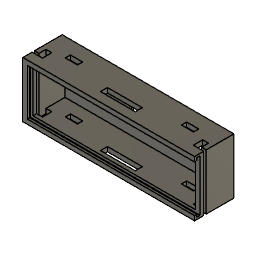
Canal - base v15 (Autodesk Fusion 360 design; units mm, degrees)
Autodesk Fusion 360 part; units mm, degrees
sketch "Esquisse1" plane through (0, 0, 0) normal (0, 1, 0) x (1, 0, 0)
  line L0 (-28.0113, -0.0987) -> (45.9887, -0.0987)
  line L1 (45.9887, -0.0987) -> (45.9887, -24.0987)
  line L2 (45.9887, -24.0987) -> (-28.0113, -24.0987)
  line L3 (-28.0113, -24.0987) -> (-28.0113, -0.0987)
  dimension "d1" = 74
  dimension "d2" = 24
  constraint horizontal L0
  constraint vertical L1
  constraint horizontal L2
  constraint vertical L3
  measures "d1" distance of L1 L3
  measures "d2" distance of L0 L2
extrude "Extrusion1" add sketch "Esquisse1" along normal blind 17
shell "Coque2" thickness 2 removed faces 1 at (21.3221, 0, 16.0987)
sketch "Esquisse3" plane through (0, 0, 0.0987) normal (0, 0, -1) x (1, 0, 0)
  line L0 (45.9887, 0) -> (-28.0113, 0)
  line L1 (-28.0113, 0) -> (-28.0113, -17)
  line L2 (-28.0113, -17) -> (45.9887, -17)
  line L3 (45.9887, -17) -> (45.9887, 0)
  line L4 (16.4887, -7) -> (1.4887, -7)
  line L5 (1.4887, -7) -> (1.4887, -4)
  line L6 (1.4887, -4) -> (16.4887, -4)
  line L7 (16.4887, -4) -> (16.4887, -7)
  line L8 (8.9887, -17) -> (8.9887, 0) construction
  dimension "d12" = 3
  dimension "d14" = 15
  dimension "d15" = 4
  constraint horizontal L4
  constraint vertical L5
  constraint horizontal L6
  constraint vertical L7
  constraint midpoint L2 L8.start
  constraint midpoint L0 L8.end
  constraint symmetric L5 L7 L8
  measures "d12" distance of L4 L6
  measures "d14" distance of L5 L7
  measures "d15" distance of L0 L6
extrude "Extrusion3" cut sketch "Esquisse3" against normal blind 25 contours L4 L5 L6 L7
sketch "Esquisse4" plane through (0, 0, 0) normal (0, 0, 1) x (1, 0, 0)
sketch "Esquisse8" plane through (0, 15, 0) normal (0, -1, 0) x (1, 0, 0)
  line L0 (43.9887, 22.0987) -> (-26.0113, 22.0987)
  line L1 (-26.0113, 22.0987) -> (-26.0113, 2.0987)
  line L2 (-26.0113, 2.0987) -> (43.9887, 2.0987)
  line L3 (43.9887, 2.0987) -> (43.9887, 22.0987)
  line L4 (-26.0113, 22.0987) -> (43.9887, 22.0987)
  line L5 (43.9887, 22.0987) -> (43.9887, 2.0987)
  line L6 (43.9887, 2.0987) -> (-26.0113, 2.0987)
  line L7 (-26.0113, 2.0987) -> (-26.0113, 22.0987)
  constraint horizontal L4
  constraint vertical L5
  constraint horizontal L6
  constraint vertical L7
  constraint coincident L2.end L3.start
  constraint coincident L0.end L1.start
extrude "Extrusion5" cut sketch "Esquisse8" against normal blind 1.2
sketch "Esquisse9" plane through (0, 17, 0) normal (0, 1, 0) x (-1, 0, 0)
  line L0 (28.0113, 24.0987) -> (-45.9887, 24.0987)
  line L1 (-45.9887, 24.0987) -> (-45.9887, 0.0987)
  line L2 (-45.9887, 0.0987) -> (28.0113, 0.0987)
  line L3 (28.0113, 0.0987) -> (28.0113, 24.0987)
  circle A0 centre (16.0113, 12.0987) radius 6.25
  circle A1 centre (-8.9887, 12.0987) radius 6.25
  circle A2 centre (-33.9887, 12.0987) radius 6.25
  dimension "d25" = 12.5
  dimension "d26" = 12
  dimension "d29" = -50
  dimension "d30" = 0
  measures "d25" diameter of A0
  measures "d26" distance of L3 A0.centre
extrude "Extrusion6" cut sketch "Esquisse9" against normal blind 1 contours A0 | A1 | A2
ref_plane "Plan de construction1" through (8.9887, 8.1, 12.0987) normal (0, 0, 1) x (1, 0, 0)
sketch "Esquisse10" plane through (0, 0, 22.0987) normal (0, 0, -1) x (1, 0, 0)
  line L0 (1.4887, -7) -> (1.4887, -4)
  line L1 (1.4887, -4) -> (16.4887, -4)
  line L2 (16.4887, -4) -> (16.4887, -7)
  line L3 (16.4887, -7) -> (1.4887, -7)
  line L4 (43.9887, 0) -> (-26.0113, 0)
  line L5 (-26.0113, 0) -> (-26.0113, -16.2)
  line L6 (-26.0113, -16.2) -> (43.9887, -16.2)
  line L7 (43.9887, -16.2) -> (43.9887, 0)
  line L8 (-18.6113, -9) -> (-13.4113, -9)
  line L9 (-13.4113, -9) -> (-13.4113, -11.2)
  line L10 (-13.4113, -11.2) -> (-18.6113, -11.2)
  line L11 (-18.6113, -11.2) -> (-18.6113, -9)
  line L12 (8.9887, 0) -> (8.9887, -15.2) construction
  line L13 (-16.0113, -9) -> (-16.0113, -11.2) construction
  line L14 (36.5887, -11.2) -> (36.5887, -9)
  line L15 (36.5887, -9) -> (31.3887, -9)
  line L16 (31.3887, -9) -> (31.3887, -11.2)
  line L17 (31.3887, -11.2) -> (36.5887, -11.2)
  dimension "d33" = 5.2
  dimension "d34" = 2.2
  dimension "d35" = 5
  dimension "d36" = 25
  constraint horizontal L8
  constraint vertical L9
  constraint horizontal L10
  constraint vertical L11
  constraint midpoint L4 L12.start
  constraint perpendicular L6 L12
  constraint midpoint L8 L13.start
  constraint midpoint L10 L13.end
  constraint symmetric L8.start L12 L14.end
  constraint symmetric L8.end L12 L15.end
  constraint symmetric L9.end L12 L16.end
  constraint symmetric L10.end L12 L14.start
  measures "d33" distance of L9 L11
  measures "d34" distance of L8 L10
  measures "d35" distance of L6 L10
  measures "d36" distance of L12 L13
extrude "Extrusion7" cut sketch "Esquisse10" against normal blind 2 contours L8 L9 L10 L11 | L14 L15 L16 L17
mirror "Symétrie miroir1" about plane through (8.9887, 8.1, 12.0987) normal (0, 0, 1) of "Extrusion7"
sketch "Esquisse11" plane through (45.9887, 0, 0) normal (1, 0, 0) x (0, 1, 0)
  line L0 (0, 24.0987) -> (0, 0.0987)
  line L1 (0, 0.0987) -> (17, 0.0987)
  line L2 (17, 0.0987) -> (17, 24.0987)
  line L3 (17, 24.0987) -> (0, 24.0987)
  line L4 (1, 23.1987) -> (2.4, 23.1987)
  line L5 (2.4, 23.1987) -> (2.4, 0.9987)
  line L6 (2.4, 0.9987) -> (1, 0.9987)
  line L7 (1, 0.9987) -> (1, 23.1987)
  line L8 (0, 12.0987) -> (17, 12.0987) construction
  dimension "d41" = 1.4
  dimension "d42" = 1
  dimension "d43" = 0.9
  constraint horizontal L4
  constraint vertical L5
  constraint horizontal L6
  constraint vertical L7
  constraint midpoint L0 L8.start
  constraint midpoint L2 L8.end
  constraint symmetric L4 L6 L8
  measures "d41" distance of L5 L7
  measures "d42" distance of L0 L7
  measures "d43" distance of L1 L6
extrude "Extrusion8" cut sketch "Esquisse11" against normal blind 73 contours L4 L5 L6 L7
sketch "Esquisse12" plane through (0, 0, 0) normal (0, -1, 0) x (1, 0, 0)
  line L0 (-26.0113, 2.0987) -> (-26.0113, 22.0987)
  line L1 (-26.0113, 22.0987) -> (43.9887, 22.0987)
  line L2 (43.9887, 22.0987) -> (43.9887, 2.0987)
  line L3 (43.9887, 2.0987) -> (-26.0113, 2.0987)
  line L4 (45.9887, 24.0987) -> (-28.0113, 24.0987)
  line L5 (-28.0113, 24.0987) -> (-28.0113, 0.0987)
  line L6 (-28.0113, 0.0987) -> (45.9887, 0.0987)
  line L7 (45.9887, 0.0987) -> (45.9887, 24.0987)
  line L8 (43.9887, 2.0987) -> (45.9887, 2.0987)
  line L9 (43.9887, 22.0987) -> (45.9887, 22.0987)
  constraint coincident L2.end L3.start
  constraint coincident L7 L8.end
  constraint perpendicular L7 L8
  constraint coincident L1.end L2.start
  constraint coincident L7 L9.end
  constraint perpendicular L7 L9
extrude "Extrusion9" cut sketch "Esquisse12" against normal blind 1 contours L2 L7 L8 L9
sketch "Esquisse15" plane through (0, 0, 0.0987) normal (0, 0, -1) x (1, 0, 0)
  line L0 (-13.4113, -9) -> (-13.4113, -11.2)
  line L1 (-13.4113, -11.2) -> (-18.6113, -11.2)
  line L2 (-18.6113, -11.2) -> (-18.6113, -9)
  line L3 (-18.6113, -9) -> (-13.4113, -9)
  line L4 (36.5887, -9) -> (36.5887, -11.2)
  line L5 (36.5887, -11.2) -> (31.3887, -11.2)
  line L6 (31.3887, -11.2) -> (31.3887, -9)
  line L7 (31.3887, -9) -> (36.5887, -9)
  line L8 (1.4887, -7) -> (1.4887, -4)
  line L9 (1.4887, -4) -> (16.4887, -4)
  line L10 (16.4887, -4) -> (16.4887, -7)
  line L11 (16.4887, -7) -> (1.4887, -7)
  line L12 (45.9887, 0) -> (-28.0113, 0)
  line L13 (-28.0113, 0) -> (-28.0113, -17)
  line L14 (-28.0113, -17) -> (45.9887, -17)
  line L15 (45.9887, -17) -> (45.9887, 0)
  line L16 (45.9887, -4) -> (41.4887, -4)
  line L17 (41.4887, -4) -> (41.4887, -8)
  line L18 (41.4887, -8) -> (43.9887, -8)
  line L19 (43.9887, -8) -> (43.9887, -5)
  line L20 (43.9887, -5) -> (45.9887, -5)
  line L21 (8.9887, 0) -> (8.9887, -17) construction
  line L22 (-26.0113, -5) -> (-28.0113, -5)
  line L23 (-26.0113, -8) -> (-26.0113, -5)
  line L24 (-23.5113, -8) -> (-26.0113, -8)
  line L25 (-23.5113, -4) -> (-23.5113, -8)
  line L26 (-28.0113, -4) -> (-23.5113, -4)
  dimension "d49" = 1
  dimension "d50" = 2
  dimension "d51" = 2.5
  dimension "d52" = 4
  dimension "d53" = 1
  constraint coincident L15 L16.start
  constraint perpendicular L15 L16
  constraint perpendicular L16 L17
  constraint perpendicular L17 L18
  constraint perpendicular L18 L19
  constraint coincident L15 L20.end
  constraint perpendicular L15 L20
  constraint midpoint L12 L21.start
  constraint midpoint L14 L21.end
  constraint symmetric L16.start L21 L26.start
  constraint symmetric L16.end L21 L25.start
  constraint symmetric L17.end L21 L24.start
  constraint symmetric L18.end L21 L23.start
  constraint symmetric L19.end L21 L22.start
  constraint symmetric L20.end L21 L22.end
  measures "d49" distance of L16 L20
  measures "d50" distance of L15 L19
  measures "d51" distance of L17 L19
  measures "d52" distance of L16 L18
  measures "d53" distance of L7 L18
extrude "Extrusion10" cut sketch "Esquisse15" against normal blind 31 contours L15 L16 L17 L18 L19 L20 | L13 L22 L23 L24 L25 L26
